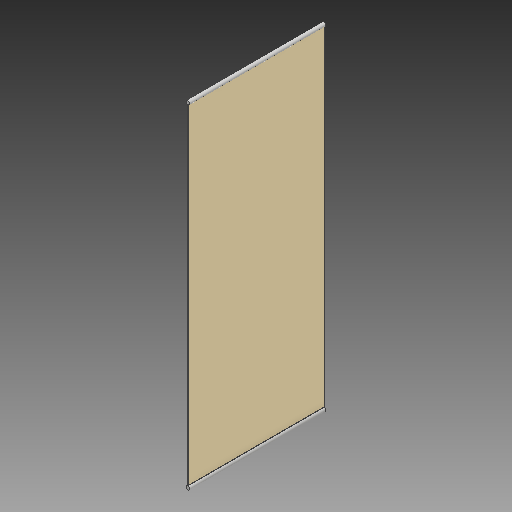
# Autodesk Inventor part: Sail
Saved by Autodesk Inventor 2018 (Build 220112000, 112)
## iProperties
Created: 2016-02-23
Part Number: Sail
Material: Generic
Document SubType Name: Modeling
Designer: Tore Den Store
Density: 1 g/cm^3
Appearance: Default
Author: Tore Den Store
Autodesk Inventor part; units mm, degrees
ref_plane "YZ Plane" through (0, 0, 0) normal (1, 0, 0) x (0, 1, 0)
ref_plane "XZ Plane" through (0, 0, 0) normal (0, 1, 0) x (-1, 0, 0)
sketch "Sketch1" plane through (0, 0, 0) normal (0, 1, 0) x (-1, 0, 0)
  circle A0 centre (0, 0) radius 10
  dimension "d0" = 20
  constraints: 1 centre point, 1 coincident
  measures "d0" diameter of A0
extrude "Extrusion1" add sketch "Sketch1" along normal blind 750
sketch "Sketch2" plane through (0, 0, 0) normal (0, -1, 0) x (1, 0, 0)
  circle A0 centre (0, 0) radius 10 projected
  line L0 (0, 10) -> (0, 1826)
  circle A1 centre (0, 1836) radius 10
  dimension "d4" = 20
  dimension "d14" = 1856
  dimension "d5" = 10
  dimension "d6" = 0
  constraints: 2 end point, 2 vertical alignment, 1 vertical, 3 other
  measures "d5" distance of L0.end point (0, 1836)
  measures "d6" distance from line of point (0, 0) L0
extrude "Extrusion2" add sketch "Sketch2" against normal blind 750 contours A1
ref_plane "Work Plane1" through (0, 0, 10) normal (0, 0, 1) x (1, 0, 0)
sketch "Sketch3" plane through (0, 0, 10) normal (0, 0, 1) x (1, 0, 0)
  line L0 (10, 750) -> (-10, 750) projected
  line L1 (-0.75, 750) -> (0.75, 750)
  line L2 (0.75, 750) -> (0.75, 0)
  line L3 (0.75, 0) -> (-0.75, 0)
  line L4 (-0.75, 0) -> (-0.75, 750)
  line L5 (10, 0) -> (10, 750) projected
  point P0 (0, 0)
  dimension "d9" = 1.5
  dimension "d10" = 750
  dimension "d11" = 9.25
  constraints: 8 end point, 2 parallel, 1 horizontal, 1 perpendicular, 1 point on line
  measures "d9" distance between parallel lines of L2 L4
  measures "d10" distance of L1.end L2.end
  measures "d11" distance between parallel lines of L5 L2
extrude "Extrusion3" add sketch "Sketch3" along normal up to surface
body "Solid1"
